Autodesk Fusion 360 part; units mm, degrees
(part 36 of 40)
  line L9834 (264.7992, 181.2097) -> (264.9001, 181.2807) construction
  line L9835 (264.9001, 181.2807) -> (265.0226, 181.3748) construction
  line L9836 (265.0226, 181.3748) -> (265.1426, 181.4727) construction
  line L9837 (265.1426, 181.4727) -> (265.2609, 181.5729) construction
  line L9838 (265.2609, 181.5729) -> (265.3784, 181.6744) construction
  line L9839 (265.3784, 181.6744) -> (265.4954, 181.7767) construction
  line L9840 (265.4954, 181.7767) -> (265.6117, 181.88) construction
  line L9841 (265.6117, 181.88) -> (265.7271, 181.9844) construction
  line L9842 (265.7271, 181.9844) -> (265.8414, 182.0903) construction
  line L9843 (265.8414, 182.0903) -> (265.9544, 182.1981) construction
  line L9844 (265.9544, 182.1981) -> (266.066, 182.3077) construction
  line L9845 (266.066, 182.3077) -> (266.1764, 182.419) construction
  line L9846 (266.1764, 182.419) -> (266.2857, 182.5316) construction
  line L9847 (266.2857, 182.5316) -> (266.3942, 182.6455) construction
  line L9848 (266.3942, 182.6455) -> (266.5018, 182.7603) construction
  line L9849 (266.5018, 182.7603) -> (266.6087, 182.876) construction
  line L9850 (266.6087, 182.876) -> (266.7148, 182.9927) construction
  line L9851 (266.7148, 182.9927) -> (266.8201, 183.1105) construction
  line L9852 (266.8201, 183.1105) -> (266.9246, 183.2292) construction
  line L9853 (266.9246, 183.2292) -> (267.0281, 183.3491) construction
  line L9854 (267.0281, 183.3491) -> (267.1308, 183.47) construction
  line L9855 (267.1308, 183.47) -> (267.2327, 183.5919) construction
  line L9856 (267.2327, 183.5919) -> (267.3337, 183.7148) construction
  line L9857 (267.3337, 183.7148) -> (267.434, 183.8386) construction
  line L9858 (267.434, 183.8386) -> (267.5335, 183.9633) construction
  line L9859 (267.5335, 183.9633) -> (267.6323, 184.0888) construction
  line L9860 (267.6323, 184.0888) -> (267.7304, 184.2151) construction
  line L9861 (267.7304, 184.2151) -> (267.8277, 184.3423) construction
  line L9862 (267.8277, 184.3423) -> (267.9243, 184.4703) construction
  line L9863 (267.9243, 184.4703) -> (268.0201, 184.5991) construction
  line L9864 (268.0201, 184.5991) -> (268.1152, 184.7288) construction
  line L9865 (268.1152, 184.7288) -> (268.2096, 184.8592) construction
  line L9866 (268.2096, 184.8592) -> (268.3032, 184.9905) construction
  line L9867 (268.3032, 184.9905) -> (268.3962, 185.1224) construction
  line L9868 (268.3962, 185.1224) -> (268.4884, 185.2552) construction
  line L9869 (268.4884, 185.2552) -> (268.58, 185.3886) construction
  line L9870 (268.58, 185.3886) -> (268.6708, 185.5228) construction
  line L9871 (268.6708, 185.5228) -> (268.761, 185.6577) construction
  line L9872 (268.761, 185.6577) -> (268.8505, 185.7933) construction
  line L9873 (268.8505, 185.7933) -> (268.9393, 185.9295) construction
  line L9874 (268.9393, 185.9295) -> (269.0275, 186.0665) construction
  line L9875 (269.0275, 186.0665) -> (269.1149, 186.2042) construction
  line L9876 (269.1149, 186.2042) -> (269.2017, 186.3425) construction
  line L9877 (269.2017, 186.3425) -> (269.2878, 186.4815) construction
  line L9878 (269.2878, 186.4815) -> (269.3733, 186.6211) construction
  line L9879 (269.3733, 186.6211) -> (269.4581, 186.7614) construction
  line L9880 (269.4581, 186.7614) -> (269.5422, 186.9023) construction
  line L9881 (269.5422, 186.9023) -> (269.6257, 187.0438) construction
  line L9882 (269.6257, 187.0438) -> (269.7085, 187.186) construction
  line L9883 (269.7085, 187.186) -> (269.7907, 187.3288) construction
  line L9884 (269.7907, 187.3288) -> (269.8723, 187.4721) construction
  line L9885 (269.8723, 187.4721) -> (269.9532, 187.6161) construction
  line L9886 (269.9532, 187.6161) -> (270.0334, 187.7607) construction
  line L9887 (270.0334, 187.7607) -> (270.113, 187.9058) construction
  line L9888 (270.113, 187.9058) -> (270.192, 188.0515) construction
  line L9889 (270.192, 188.0515) -> (270.2703, 188.1978) construction
  line L9890 (270.2703, 188.1978) -> (270.348, 188.3447) construction
  line L9891 (270.348, 188.3447) -> (270.4251, 188.4921) construction
  line L9892 (270.4251, 188.4921) -> (270.5015, 188.6401) construction
  line L9893 (270.5015, 188.6401) -> (270.5773, 188.7886) construction
  line L9894 (270.5773, 188.7886) -> (270.6525, 188.9377) construction
  line L9895 (270.6525, 188.9377) -> (270.727, 189.0873) construction
  line L9896 (270.727, 189.0873) -> (270.801, 189.2374) construction
  line L9897 (270.801, 189.2374) -> (270.8743, 189.3881) construction
  line L9898 (270.8743, 189.3881) -> (270.9469, 189.5393) construction
  line L9899 (270.9469, 189.5393) -> (271.019, 189.6909) construction
  line L9900 (271.019, 189.6909) -> (271.0904, 189.8431) construction
  line L9901 (271.0904, 189.8431) -> (271.1471, 189.9653) construction
  line L9902 (271.1471, 189.9653) -> (271.1893, 190.0572) construction
  line L9903 (271.1893, 190.0572) -> (271.2173, 190.1185) construction
  line L9904 (271.2173, 190.1185) -> (271.2313, 190.1492) construction
  arc A254 (283.5435, 147.7437) -> (283.5435, 152.2563) centre (212.132, 150) ccw
  spline S132 degree 5 poles (257.9473, 109.6737) (257.9705, 109.6533) (258.0174, 109.6132) (258.0893, 109.5549) (258.188, 109.4808) (258.3153, 109.3934) (258.4455, 109.3096) (258.5774, 109.228) (258.7102, 109.1476) (258.8437, 109.068) (258.9778, 108.9893) (259.1127, 108.9117) (259.2488, 108.8358) (259.3863, 108.7617) (259.525, 108.6894) (259.6649, 108.6187) (259.8058, 108.5496) (259.9476, 108.4816) (260.0901, 108.4147) (260.2332, 108.3488) (260.377, 108.284) (260.5215, 108.2202) (260.6667, 108.1576) (260.8127, 108.0961) (260.9594, 108.0358) (261.1069, 107.9766) (261.255, 107.9185) (261.4037, 107.8614) (261.553, 107.8053) (261.7029, 107.7501) (261.8534, 107.6959) (262.0044, 107.6426) (262.156, 107.5903) (262.3081, 107.539) (262.4608, 107.4886) (262.614, 107.4392) (262.7678, 107.3906) (262.922, 107.343) (263.0767, 107.2963) (263.2319, 107.2505) (263.3876, 107.2055) (263.5438, 107.1614) (263.7004, 107.1182) (263.8575, 107.0759) (264.015, 107.0344) (264.1729, 106.9937) (264.3313, 106.9539) (264.4901, 106.915) (264.6493, 106.8769) (264.8089, 106.8396) (264.9689, 106.8031) (265.1293, 106.7674) (265.2901, 106.7326) (265.4513, 106.6985) (265.6129, 106.6653) (265.7748, 106.6328) (265.9371, 106.6012) (266.0997, 106.5703) (266.2627, 106.5403) (266.426, 106.511) (266.5897, 106.4825) (266.7537, 106.4547) (266.9181, 106.4277) (267.0828, 106.4016) (267.2478, 106.3761) (267.4131, 106.3514) (267.5787, 106.3275) (267.7446, 106.3044) (267.9109, 106.282) (268.0774, 106.2603) (268.2442, 106.2394) (268.3779, 106.2233) (268.4783, 106.2115) (268.5453, 106.2038) (268.5789, 106.2) knots 0 0 0 0 0 0 0.01428571 0.02857143 0.04285714 0.05714286 0.07142857 0.08571429 0.1 0.11428571 0.12857143 0.14285714 0.15714286 0.17142857 0.18571429 0.2 0.21428571 0.22857143 0.24285714 0.25714286 0.27142857 0.28571429 0.3 0.31428571 0.32857143 0.34285714 0.35714286 0.37142857 0.38571429 0.4 0.41428571 0.42857143 0.44285714 0.45714286 0.47142857 0.48571429 0.5 0.51428571 0.52857143 0.54285714 0.55714286 0.57142857 0.58571429 0.6 0.61428571 0.62857143 0.64285714 0.65714286 0.67142857 0.68571429 0.7 0.71428571 0.72857143 0.74285714 0.75714286 0.77142857 0.78571429 0.8 0.81428571 0.82857143 0.84285714 0.85714286 0.87142857 0.88571429 0.9 0.91428571 0.92857143 0.94285714 0.95714286 0.97142857 0.98571429 1 1 1 1 1 1
  line L9905 (257.9473, 109.6737) -> (257.9705, 109.6533) construction
  line L9906 (257.9705, 109.6533) -> (258.0174, 109.6132) construction
  line L9907 (258.0174, 109.6132) -> (258.0893, 109.5549) construction
  line L9908 (258.0893, 109.5549) -> (258.188, 109.4808) construction
  line L9909 (258.188, 109.4808) -> (258.3153, 109.3934) construction
  line L9910 (258.3153, 109.3934) -> (258.4455, 109.3096) construction
  line L9911 (258.4455, 109.3096) -> (258.5774, 109.228) construction
  line L9912 (258.5774, 109.228) -> (258.7102, 109.1476) construction
  line L9913 (258.7102, 109.1476) -> (258.8437, 109.068) construction
  line L9914 (258.8437, 109.068) -> (258.9778, 108.9893) construction
  line L9915 (258.9778, 108.9893) -> (259.1127, 108.9117) construction
  line L9916 (259.1127, 108.9117) -> (259.2488, 108.8358) construction
  line L9917 (259.2488, 108.8358) -> (259.3863, 108.7617) construction
  line L9918 (259.3863, 108.7617) -> (259.525, 108.6894) construction
  line L9919 (259.525, 108.6894) -> (259.6649, 108.6187) construction
  line L9920 (259.6649, 108.6187) -> (259.8058, 108.5496) construction
  line L9921 (259.8058, 108.5496) -> (259.9476, 108.4816) construction
  line L9922 (259.9476, 108.4816) -> (260.0901, 108.4147) construction
  line L9923 (260.0901, 108.4147) -> (260.2332, 108.3488) construction
  line L9924 (260.2332, 108.3488) -> (260.377, 108.284) construction
  line L9925 (260.377, 108.284) -> (260.5215, 108.2202) construction
  line L9926 (260.5215, 108.2202) -> (260.6667, 108.1576) construction
  line L9927 (260.6667, 108.1576) -> (260.8127, 108.0961) construction
  line L9928 (260.8127, 108.0961) -> (260.9594, 108.0358) construction
  line L9929 (260.9594, 108.0358) -> (261.1069, 107.9766) construction
  line L9930 (261.1069, 107.9766) -> (261.255, 107.9185) construction
  line L9931 (261.255, 107.9185) -> (261.4037, 107.8614) construction
  line L9932 (261.4037, 107.8614) -> (261.553, 107.8053) construction
  line L9933 (261.553, 107.8053) -> (261.7029, 107.7501) construction
  line L9934 (261.7029, 107.7501) -> (261.8534, 107.6959) construction
  line L9935 (261.8534, 107.6959) -> (262.0044, 107.6426) construction
  line L9936 (262.0044, 107.6426) -> (262.156, 107.5903) construction
  line L9937 (262.156, 107.5903) -> (262.3081, 107.539) construction
  line L9938 (262.3081, 107.539) -> (262.4608, 107.4886) construction
  line L9939 (262.4608, 107.4886) -> (262.614, 107.4392) construction
  line L9940 (262.614, 107.4392) -> (262.7678, 107.3906) construction
  line L9941 (262.7678, 107.3906) -> (262.922, 107.343) construction
  line L9942 (262.922, 107.343) -> (263.0767, 107.2963) construction
  line L9943 (263.0767, 107.2963) -> (263.2319, 107.2505) construction
  line L9944 (263.2319, 107.2505) -> (263.3876, 107.2055) construction
  line L9945 (263.3876, 107.2055) -> (263.5438, 107.1614) construction
  line L9946 (263.5438, 107.1614) -> (263.7004, 107.1182) construction
  line L9947 (263.7004, 107.1182) -> (263.8575, 107.0759) construction
  line L9948 (263.8575, 107.0759) -> (264.015, 107.0344) construction
  line L9949 (264.015, 107.0344) -> (264.1729, 106.9937) construction
  line L9950 (264.1729, 106.9937) -> (264.3313, 106.9539) construction
  line L9951 (264.3313, 106.9539) -> (264.4901, 106.915) construction
  line L9952 (264.4901, 106.915) -> (264.6493, 106.8769) construction
  line L9953 (264.6493, 106.8769) -> (264.8089, 106.8396) construction
  line L9954 (264.8089, 106.8396) -> (264.9689, 106.8031) construction
  line L9955 (264.9689, 106.8031) -> (265.1293, 106.7674) construction
  line L9956 (265.1293, 106.7674) -> (265.2901, 106.7326) construction
  line L9957 (265.2901, 106.7326) -> (265.4513, 106.6985) construction
  line L9958 (265.4513, 106.6985) -> (265.6129, 106.6653) construction
  line L9959 (265.6129, 106.6653) -> (265.7748, 106.6328) construction
  line L9960 (265.7748, 106.6328) -> (265.9371, 106.6012) construction
  line L9961 (265.9371, 106.6012) -> (266.0997, 106.5703) construction
  line L9962 (266.0997, 106.5703) -> (266.2627, 106.5403) construction
  line L9963 (266.2627, 106.5403) -> (266.426, 106.511) construction
  line L9964 (266.426, 106.511) -> (266.5897, 106.4825) construction
  line L9965 (266.5897, 106.4825) -> (266.7537, 106.4547) construction
  line L9966 (266.7537, 106.4547) -> (266.9181, 106.4277) construction
  line L9967 (266.9181, 106.4277) -> (267.0828, 106.4016) construction
  line L9968 (267.0828, 106.4016) -> (267.2478, 106.3761) construction
  line L9969 (267.2478, 106.3761) -> (267.4131, 106.3514) construction
  line L9970 (267.4131, 106.3514) -> (267.5787, 106.3275) construction
  line L9971 (267.5787, 106.3275) -> (267.7446, 106.3044) construction
  line L9972 (267.7446, 106.3044) -> (267.9109, 106.282) construction
  line L9973 (267.9109, 106.282) -> (268.0774, 106.2603) construction
  line L9974 (268.0774, 106.2603) -> (268.2442, 106.2394) construction
  line L9975 (268.2442, 106.2394) -> (268.3779, 106.2233) construction
  line L9976 (268.3779, 106.2233) -> (268.4783, 106.2115) construction
  line L9977 (268.4783, 106.2115) -> (268.5453, 106.2038) construction
  line L9978 (268.5453, 106.2038) -> (268.5789, 106.2) construction
  arc A255 (155.1583, 142.7194) -> (155.697, 139.3184) centre (212.132, 150) ccw
  arc A256 (204.8514, 206.9737) -> (201.4504, 206.435) centre (212.132, 150) ccw
  arc A257 (219.4126, 93.0263) -> (222.8136, 93.565) centre (212.132, 150) ccw
  arc A258 (219.4126, 93.0263) -> (217.6748, 90.8558) centre (219.6661, 91.0425) ccw
  arc A259 (172.7536, 191.8132) -> (170.3188, 189.3784) centre (212.132, 150) ccw
  spline S133 degree 5 poles (206.4369, 89.2315) (206.4341, 89.2007) (206.4291, 89.1391) (206.4242, 89.0467) (206.4223, 88.9234) (206.4264, 88.769) (206.4351, 88.6144) (206.4466, 88.4597) (206.4597, 88.305) (206.4737, 88.1502) (206.4889, 87.9955) (206.5055, 87.8407) (206.524, 87.686) (206.5449, 87.5312) (206.5679, 87.3765) (206.593, 87.2218) (206.6199, 87.0671) (206.6482, 86.9125) (206.6778, 86.7579) (206.7087, 86.6034) (206.7407, 86.4489) (206.7741, 86.2945) (206.8088, 86.1402) (206.8449, 85.986) (206.8823, 85.8318) (206.9211, 85.6778) (206.9611, 85.5238) (207.0023, 85.3699) (207.0447, 85.2161) (207.0881, 85.0624) (207.1327, 84.9088) (207.1784, 84.7553) (207.2252, 84.602) (207.2731, 84.4487) (207.3221, 84.2956) (207.3721, 84.1426) (207.4233, 83.9897) (207.4754, 83.8369) (207.5285, 83.6842) (207.5827, 83.5317) (207.6378, 83.3794) (207.694, 83.2271) (207.751, 83.075) (207.8091, 82.923) (207.8681, 82.7712) (207.9281, 82.6196) (207.989, 82.468) (208.0508, 82.3167) (208.1135, 82.1655) (208.1772, 82.0144) (208.2417, 81.8635) (208.3071, 81.7128) (208.3735, 81.5622) (208.4407, 81.4118) (208.5087, 81.2616) (208.5777, 81.1115) (208.6474, 80.9616) (208.7181, 80.8119) (208.7895, 80.6624) (208.8619, 80.513) (208.935, 80.3638) (209.009, 80.2148) (209.0838, 80.066) (209.1594, 79.9174) (209.2358, 79.7689) (209.313, 79.6207) (209.391, 79.4726) (209.4698, 79.3248) (209.5494, 79.1771) (209.6297, 79.0297) (209.7109, 78.8824) (209.7764, 78.7648) (209.8259, 78.6766) (209.8591, 78.6179) (209.8757, 78.5885) knots 0 0 0 0 0 0 0.01428571 0.02857143 0.04285714 0.05714286 0.07142857 0.08571429 0.1 0.11428571 0.12857143 0.14285714 0.15714286 0.17142857 0.18571429 0.2 0.21428571 0.22857143 0.24285714 0.25714286 0.27142857 0.28571429 0.3 0.31428571 0.32857143 0.34285714 0.35714286 0.37142857 0.38571429 0.4 0.41428571 0.42857143 0.44285714 0.45714286 0.47142857 0.48571429 0.5 0.51428571 0.52857143 0.54285714 0.55714286 0.57142857 0.58571429 0.6 0.61428571 0.62857143 0.64285714 0.65714286 0.67142857 0.68571429 0.7 0.71428571 0.72857143 0.74285714 0.75714286 0.77142857 0.78571429 0.8 0.81428571 0.82857143 0.84285714 0.85714286 0.87142857 0.88571429 0.9 0.91428571 0.92857143 0.94285714 0.95714286 0.97142857 0.98571429 1 1 1 1 1 1
  line L9979 (206.4369, 89.2315) -> (206.4341, 89.2007) construction
  line L9980 (206.4341, 89.2007) -> (206.4291, 89.1391) construction
  line L9981 (206.4291, 89.1391) -> (206.4242, 89.0467) construction
  line L9982 (206.4242, 89.0467) -> (206.4223, 88.9234) construction
  line L9983 (206.4223, 88.9234) -> (206.4264, 88.769) construction
  line L9984 (206.4264, 88.769) -> (206.4351, 88.6144) construction
  line L9985 (206.4351, 88.6144) -> (206.4466, 88.4597) construction
  line L9986 (206.4466, 88.4597) -> (206.4597, 88.305) construction
  line L9987 (206.4597, 88.305) -> (206.4737, 88.1502) construction
  line L9988 (206.4737, 88.1502) -> (206.4889, 87.9955) construction
  line L9989 (206.4889, 87.9955) -> (206.5055, 87.8407) construction
  line L9990 (206.5055, 87.8407) -> (206.524, 87.686) construction
  line L9991 (206.524, 87.686) -> (206.5449, 87.5312) construction
  line L9992 (206.5449, 87.5312) -> (206.5679, 87.3765) construction
  line L9993 (206.5679, 87.3765) -> (206.593, 87.2218) construction
  line L9994 (206.593, 87.2218) -> (206.6199, 87.0671) construction
  line L9995 (206.6199, 87.0671) -> (206.6482, 86.9125) construction
  line L9996 (206.6482, 86.9125) -> (206.6778, 86.7579) construction
  line L9997 (206.6778, 86.7579) -> (206.7087, 86.6034) construction
  line L9998 (206.7087, 86.6034) -> (206.7407, 86.4489) construction
  line L9999 (206.7407, 86.4489) -> (206.7741, 86.2945) construction
  line L10000 (206.7741, 86.2945) -> (206.8088, 86.1402) construction
  line L10001 (206.8088, 86.1402) -> (206.8449, 85.986) construction
  line L10002 (206.8449, 85.986) -> (206.8823, 85.8318) construction
  line L10003 (206.8823, 85.8318) -> (206.9211, 85.6778) construction
  line L10004 (206.9211, 85.6778) -> (206.9611, 85.5238) construction
  line L10005 (206.9611, 85.5238) -> (207.0023, 85.3699) construction
  line L10006 (207.0023, 85.3699) -> (207.0447, 85.2161) construction
  line L10007 (207.0447, 85.2161) -> (207.0881, 85.0624) construction
  line L10008 (207.0881, 85.0624) -> (207.1327, 84.9088) construction
  line L10009 (207.1327, 84.9088) -> (207.1784, 84.7553) construction
  line L10010 (207.1784, 84.7553) -> (207.2252, 84.602) construction
  line L10011 (207.2252, 84.602) -> (207.2731, 84.4487) construction
  line L10012 (207.2731, 84.4487) -> (207.3221, 84.2956) construction
  line L10013 (207.3221, 84.2956) -> (207.3721, 84.1426) construction
  line L10014 (207.3721, 84.1426) -> (207.4233, 83.9897) construction
  line L10015 (207.4233, 83.9897) -> (207.4754, 83.8369) construction
  line L10016 (207.4754, 83.8369) -> (207.5285, 83.6842) construction
  line L10017 (207.5285, 83.6842) -> (207.5827, 83.5317) construction
  line L10018 (207.5827, 83.5317) -> (207.6378, 83.3794) construction
  line L10019 (207.6378, 83.3794) -> (207.694, 83.2271) construction
  line L10020 (207.694, 83.2271) -> (207.751, 83.075) construction
  line L10021 (207.751, 83.075) -> (207.8091, 82.923) construction
  line L10022 (207.8091, 82.923) -> (207.8681, 82.7712) construction
  line L10023 (207.8681, 82.7712) -> (207.9281, 82.6196) construction
  line L10024 (207.9281, 82.6196) -> (207.989, 82.468) construction
  line L10025 (207.989, 82.468) -> (208.0508, 82.3167) construction
  line L10026 (208.0508, 82.3167) -> (208.1135, 82.1655) construction
  line L10027 (208.1135, 82.1655) -> (208.1772, 82.0144) construction
  line L10028 (208.1772, 82.0144) -> (208.2417, 81.8635) construction
  line L10029 (208.2417, 81.8635) -> (208.3071, 81.7128) construction
  line L10030 (208.3071, 81.7128) -> (208.3735, 81.5622) construction
  line L10031 (208.3735, 81.5622) -> (208.4407, 81.4118) construction
  line L10032 (208.4407, 81.4118) -> (208.5087, 81.2616) construction
  line L10033 (208.5087, 81.2616) -> (208.5777, 81.1115) construction
  line L10034 (208.5777, 81.1115) -> (208.6474, 80.9616) construction
  line L10035 (208.6474, 80.9616) -> (208.7181, 80.8119) construction
  line L10036 (208.7181, 80.8119) -> (208.7895, 80.6624) construction
  line L10037 (208.7895, 80.6624) -> (208.8619, 80.513) construction
  line L10038 (208.8619, 80.513) -> (208.935, 80.3638) construction
  line L10039 (208.935, 80.3638) -> (209.009, 80.2148) construction
  line L10040 (209.009, 80.2148) -> (209.0838, 80.066) construction
  line L10041 (209.0838, 80.066) -> (209.1594, 79.9174) construction
  line L10042 (209.1594, 79.9174) -> (209.2358, 79.7689) construction
  line L10043 (209.2358, 79.7689) -> (209.313, 79.6207) construction
  line L10044 (209.313, 79.6207) -> (209.391, 79.4726) construction
  line L10045 (209.391, 79.4726) -> (209.4698, 79.3248) construction
  line L10046 (209.4698, 79.3248) -> (209.5494, 79.1771) construction
  line L10047 (209.5494, 79.1771) -> (209.6297, 79.0297) construction
  line L10048 (209.6297, 79.0297) -> (209.7109, 78.8824) construction
  line L10049 (209.7109, 78.8824) -> (209.7764, 78.7648) construction
  line L10050 (209.7764, 78.7648) -> (209.8259, 78.6766) construction
  line L10051 (209.8259, 78.6766) -> (209.8591, 78.6179) construction
  line L10052 (209.8591, 78.6179) -> (209.8757, 78.5885) construction
  arc A260 (187.6019, 201.9354) -> (188.5839, 204.5366) centre (186.7478, 203.7438) ccw
  arc A261 (239.7302, 200.3721) -> (236.6621, 201.9354) centre (212.132, 150) ccw
  spline S134 degree 5 poles (243.2435, 97.4897) (243.2592, 97.4632) (243.2914, 97.4105) (243.3417, 97.3328) (243.4127, 97.2319) (243.5068, 97.1094) (243.6047, 96.9894) (243.7049, 96.8711) (243.8064, 96.7536) (243.9087, 96.6366) (244.012, 96.5203) (244.1164, 96.4049) (244.2223, 96.2906) (244.3301, 96.1776) (244.4397, 96.066) (244.551, 95.9556) (244.6636, 95.8463) (244.7775, 95.7378) (244.8923, 95.6302) (245.008, 95.5233) (245.1247, 95.4172) (245.2425, 95.3119) (245.3612, 95.2074) (245.4811, 95.1039) (245.602, 95.0012) (245.7239, 94.8993) (245.8468, 94.7983) (245.9706, 94.698) (246.0953, 94.5985) (246.2208, 94.4997) (246.3471, 94.4016) (246.4743, 94.3043) (246.6023, 94.2077) (246.7311, 94.1119) (246.8608, 94.0168) (246.9912, 93.9224) (247.1225, 93.8288) (247.2544, 93.7358) (247.3872, 93.6436) (247.5206, 93.552) (247.6548, 93.4612) (247.7897, 93.371) (247.9253, 93.2815) (248.0615, 93.1927) (248.1985, 93.1045) (248.3362, 93.0171) (248.4745, 92.9303) (248.6135, 92.8442) (248.7531, 92.7587) (248.8934, 92.6739) (249.0343, 92.5898) (249.1758, 92.5063) (249.318, 92.4235) (249.4608, 92.3413) (249.6041, 92.2597) (249.7481, 92.1788) (249.8927, 92.0986) (250.0378, 92.019) (250.1835, 91.94) (250.3298, 91.8617) (250.4767, 91.784) (250.6241, 91.7069) (250.7721, 91.6305) (250.9206, 91.5547) (251.0697, 91.4795) (251.2193, 91.405) (251.3694, 91.331) (251.5201, 91.2577) (251.6713, 91.1851) (251.8229, 91.113) (251.9751, 91.0416) (252.0973, 90.9849) (252.1892, 90.9427) (252.2505, 90.9147) (252.2812, 90.9007) knots 0 0 0 0 0 0 0.01428571 0.02857143 0.04285714 0.05714286 0.07142857 0.08571429 0.1 0.11428571 0.12857143 0.14285714 0.15714286 0.17142857 0.18571429 0.2 0.21428571 0.22857143 0.24285714 0.25714286 0.27142857 0.28571429 0.3 0.31428571 0.32857143 0.34285714 0.35714286 0.37142857 0.38571429 0.4 0.41428571 0.42857143 0.44285714 0.45714286 0.47142857 0.48571429 0.5 0.51428571 0.52857143 0.54285714 0.55714286 0.57142857 0.58571429 0.6 0.61428571 0.62857143 0.64285714 0.65714286 0.67142857 0.68571429 0.7 0.71428571 0.72857143 0.74285714 0.75714286 0.77142857 0.78571429 0.8 0.81428571 0.82857143 0.84285714 0.85714286 0.87142857 0.88571429 0.9 0.91428571 0.92857143 0.94285714 0.95714286 0.97142857 0.98571429 1 1 1 1 1 1
  line L10053 (243.2435, 97.4897) -> (243.2592, 97.4632) construction
  line L10054 (243.2592, 97.4632) -> (243.2914, 97.4105) construction
  line L10055 (243.2914, 97.4105) -> (243.3417, 97.3328) construction
  line L10056 (243.3417, 97.3328) -> (243.4127, 97.2319) construction
  line L10057 (243.4127, 97.2319) -> (243.5068, 97.1094) construction
  line L10058 (243.5068, 97.1094) -> (243.6047, 96.9894) construction
  line L10059 (243.6047, 96.9894) -> (243.7049, 96.8711) construction
  line L10060 (243.7049, 96.8711) -> (243.8064, 96.7536) construction
  line L10061 (243.8064, 96.7536) -> (243.9087, 96.6366) construction
  line L10062 (243.9087, 96.6366) -> (244.012, 96.5203) construction
  line L10063 (244.012, 96.5203) -> (244.1164, 96.4049) construction
  line L10064 (244.1164, 96.4049) -> (244.2223, 96.2906) construction
  line L10065 (244.2223, 96.2906) -> (244.3301, 96.1776) construction
  line L10066 (244.3301, 96.1776) -> (244.4397, 96.066) construction
  line L10067 (244.4397, 96.066) -> (244.551, 95.9556) construction
  line L10068 (244.551, 95.9556) -> (244.6636, 95.8463) construction
  line L10069 (244.6636, 95.8463) -> (244.7775, 95.7378) construction
  line L10070 (244.7775, 95.7378) -> (244.8923, 95.6302) construction
  line L10071 (244.8923, 95.6302) -> (245.008, 95.5233) construction
  line L10072 (245.008, 95.5233) -> (245.1247, 95.4172) construction
  line L10073 (245.1247, 95.4172) -> (245.2425, 95.3119) construction
  line L10074 (245.2425, 95.3119) -> (245.3612, 95.2074) construction
  line L10075 (245.3612, 95.2074) -> (245.4811, 95.1039) construction
  line L10076 (245.4811, 95.1039) -> (245.602, 95.0012) construction
  line L10077 (245.602, 95.0012) -> (245.7239, 94.8993) construction
  line L10078 (245.7239, 94.8993) -> (245.8468, 94.7983) construction
  line L10079 (245.8468, 94.7983) -> (245.9706, 94.698) construction
  line L10080 (245.9706, 94.698) -> (246.0953, 94.5985) construction
  line L10081 (246.0953, 94.5985) -> (246.2208, 94.4997) construction
  line L10082 (246.2208, 94.4997) -> (246.3471, 94.4016) construction
  line L10083 (246.3471, 94.4016) -> (246.4743, 94.3043) construction
  line L10084 (246.4743, 94.3043) -> (246.6023, 94.2077) construction
  line L10085 (246.6023, 94.2077) -> (246.7311, 94.1119) construction
  line L10086 (246.7311, 94.1119) -> (246.8608, 94.0168) construction
  line L10087 (246.8608, 94.0168) -> (246.9912, 93.9224) construction
  line L10088 (246.9912, 93.9224) -> (247.1225, 93.8288) construction
  line L10089 (247.1225, 93.8288) -> (247.2544, 93.7358) construction
  line L10090 (247.2544, 93.7358) -> (247.3872, 93.6436) construction
  line L10091 (247.3872, 93.6436) -> (247.5206, 93.552) construction
  line L10092 (247.5206, 93.552) -> (247.6548, 93.4612) construction
  line L10093 (247.6548, 93.4612) -> (247.7897, 93.371) construction
  line L10094 (247.7897, 93.371) -> (247.9253, 93.2815) construction
  line L10095 (247.9253, 93.2815) -> (248.0615, 93.1927) construction
  line L10096 (248.0615, 93.1927) -> (248.1985, 93.1045) construction
  line L10097 (248.1985, 93.1045) -> (248.3362, 93.0171) construction
  line L10098 (248.3362, 93.0171) -> (248.4745, 92.9303) construction
  line L10099 (248.4745, 92.9303) -> (248.6135, 92.8442) construction
  line L10100 (248.6135, 92.8442) -> (248.7531, 92.7587) construction
  line L10101 (248.7531, 92.7587) -> (248.8934, 92.6739) construction
  line L10102 (248.8934, 92.6739) -> (249.0343, 92.5898) construction
  line L10103 (249.0343, 92.5898) -> (249.1758, 92.5063) construction
  line L10104 (249.1758, 92.5063) -> (249.318, 92.4235) construction
  line L10105 (249.318, 92.4235) -> (249.4608, 92.3413) construction
  line L10106 (249.4608, 92.3413) -> (249.6041, 92.2597) construction
  line L10107 (249.6041, 92.2597) -> (249.7481, 92.1788) construction
  line L10108 (249.7481, 92.1788) -> (249.8927, 92.0986) construction
  line L10109 (249.8927, 92.0986) -> (250.0378, 92.019) construction
  line L10110 (250.0378, 92.019) -> (250.1835, 91.94) construction
  line L10111 (250.1835, 91.94) -> (250.3298, 91.8617) construction
  line L10112 (250.3298, 91.8617) -> (250.4767, 91.784) construction
  line L10113 (250.4767, 91.784) -> (250.6241, 91.7069) construction
  line L10114 (250.6241, 91.7069) -> (250.7721, 91.6305) construction
  line L10115 (250.7721, 91.6305) -> (250.9206, 91.5547) construction
  line L10116 (250.9206, 91.5547) -> (251.0697, 91.4795) construction
  line L10117 (251.0697, 91.4795) -> (251.2193, 91.405) construction
  line L10118 (251.2193, 91.405) -> (251.3694, 91.331) construction
  line L10119 (251.3694, 91.331) -> (251.5201, 91.2577) construction
  line L10120 (251.5201, 91.2577) -> (251.6713, 91.1851) construction
  line L10121 (251.6713, 91.1851) -> (251.8229, 91.113) construction
  line L10122 (251.8229, 91.113) -> (251.9751, 91.0416) construction
  line L10123 (251.9751, 91.0416) -> (252.0973, 90.9849) construction
  line L10124 (252.0973, 90.9849) -> (252.1892, 90.9427) construction
  line L10125 (252.1892, 90.9427) -> (252.2505, 90.9147) construction
  line L10126 (252.2505, 90.9147) -> (252.2812, 90.9007) construction
  spline S135 degree 5 poles (152.5778, 136.6378) (152.5477, 136.631) (152.4876, 136.6167) (152.3982, 136.5929) (152.2803, 136.5565) (152.1347, 136.5049) (151.9904, 136.4489) (151.8468, 136.3901) (151.7037, 136.3299) (151.5609, 136.2687) (151.4184, 136.2065) (151.2763, 136.1429) (151.1349, 136.0774) (150.9941, 136.0098) (150.8541, 135.94) (150.7147, 135.8684) (150.5759, 135.795) (150.4376, 135.7203) (150.2998, 135.6443) (150.1623, 135.5673) (150.0253, 135.4891) (149.8888, 135.4096) (149.7528, 135.3289) (149.6172, 135.247) (149.4822, 135.1637) (149.3477, 135.0792) (149.2136, 134.9936) (149.08, 134.9068) (148.9468, 134.819) (148.814, 134.7302) (148.6817, 134.6403) (148.5499, 134.5494) (148.4185, 134.4575) (148.2875, 134.3646) (148.157, 134.2707) (148.027, 134.1758) (147.8974, 134.08) (147.7682, 133.9832) (147.6394, 133.8854) (147.5111, 133.7868) (147.3832, 133.6873) (147.2558, 133.5869) (147.1288, 133.4856) (147.0022, 133.3834) (146.876, 133.2804) (146.7503, 133.1765) (146.625, 133.0717) (146.5002, 132.9662) (146.3758, 132.8598) (146.2518, 132.7526) (146.1282, 132.6445) (146.0051, 132.5357) (145.8823, 132.4261) (145.7601, 132.3158) (145.6382, 132.2046) (145.5168, 132.0927) (145.3958, 131.98) (145.2752, 131.8665) (145.1551, 131.7523) (145.0354, 131.6374) (144.9161, 131.5218) (144.7973, 131.4054) (144.6789, 131.2882) (144.5609, 131.1704) (144.4433, 131.0519) (144.3262, 130.9326) (144.2095, 130.8127) (144.0932, 130.6921) (143.9774, 130.5707) (143.862, 130.4488) (143.747, 130.3261) (143.6553, 130.2274) (143.5868, 130.1531) (143.5412, 130.1034) (143.5184, 130.0785) knots 0 0 0 0 0 0 0.01428571 0.02857143 0.04285714 0.05714286 0.07142857 0.08571429 0.1 0.11428571 0.12857143 0.14285714 0.15714286 0.17142857 0.18571429 0.2 0.21428571 0.22857143 0.24285714 0.25714286 0.27142857 0.28571429 0.3 0.31428571 0.32857143 0.34285714 0.35714286 0.37142857 0.38571429 0.4 0.41428571 0.42857143 0.44285714 0.45714286 0.47142857 0.48571429 0.5 0.51428571 0.52857143 0.54285714 0.55714286 0.57142857 0.58571429 0.6 0.61428571 0.62857143 0.64285714 0.65714286 0.67142857 0.68571429 0.7 0.71428571 0.72857143 0.74285714 0.75714286 0.77142857 0.78571429 0.8 0.81428571 0.82857143 0.84285714 0.85714286 0.87142857 0.88571429 0.9 0.91428571 0.92857143 0.94285714 0.95714286 0.97142857 0.98571429 1 1 1 1 1 1
  line L10127 (152.5778, 136.6378) -> (152.5477, 136.631) construction
  line L10128 (152.5477, 136.631) -> (152.4876, 136.6167) construction
  line L10129 (152.4876, 136.6167) -> (152.3982, 136.5929) construction
  line L10130 (152.3982, 136.5929) -> (152.2803, 136.5565) construction
  line L10131 (152.2803, 136.5565) -> (152.1347, 136.5049) construction
  line L10132 (152.1347, 136.5049) -> (151.9904, 136.4489) construction
  line L10133 (151.9904, 136.4489) -> (151.8468, 136.3901) construction
  line L10134 (151.8468, 136.3901) -> (151.7037, 136.3299) construction
  line L10135 (151.7037, 136.3299) -> (151.5609, 136.2687) construction
  line L10136 (151.5609, 136.2687) -> (151.4184, 136.2065) construction
  line L10137 (151.4184, 136.2065) -> (151.2763, 136.1429) construction
  line L10138 (151.2763, 136.1429) -> (151.1349, 136.0774) construction
  line L10139 (151.1349, 136.0774) -> (150.9941, 136.0098) construction
  line L10140 (150.9941, 136.0098) -> (150.8541, 135.94) construction
  line L10141 (150.8541, 135.94) -> (150.7147, 135.8684) construction
  line L10142 (150.7147, 135.8684) -> (150.5759, 135.795) construction
  line L10143 (150.5759, 135.795) -> (150.4376, 135.7203) construction
  line L10144 (150.4376, 135.7203) -> (150.2998, 135.6443) construction
  line L10145 (150.2998, 135.6443) -> (150.1623, 135.5673) construction
  line L10146 (150.1623, 135.5673) -> (150.0253, 135.4891) construction
  line L10147 (150.0253, 135.4891) -> (149.8888, 135.4096) construction
  line L10148 (149.8888, 135.4096) -> (149.7528, 135.3289) construction
  line L10149 (149.7528, 135.3289) -> (149.6172, 135.247) construction
  line L10150 (149.6172, 135.247) -> (149.4822, 135.1637) construction
  line L10151 (149.4822, 135.1637) -> (149.3477, 135.0792) construction
  line L10152 (149.3477, 135.0792) -> (149.2136, 134.9936) construction
  line L10153 (149.2136, 134.9936) -> (149.08, 134.9068) construction
  line L10154 (149.08, 134.9068) -> (148.9468, 134.819) construction
  line L10155 (148.9468, 134.819) -> (148.814, 134.7302) construction
  line L10156 (148.814, 134.7302) -> (148.6817, 134.6403) construction
  line L10157 (148.6817, 134.6403) -> (148.5499, 134.5494) construction
  line L10158 (148.5499, 134.5494) -> (148.4185, 134.4575) construction
  line L10159 (148.4185, 134.4575) -> (148.2875, 134.3646) construction
  line L10160 (148.2875, 134.3646) -> (148.157, 134.2707) construction
  line L10161 (148.157, 134.2707) -> (148.027, 134.1758) construction
  line L10162 (148.027, 134.1758) -> (147.8974, 134.08) construction
  line L10163 (147.8974, 134.08) -> (147.7682, 133.9832) construction
  line L10164 (147.7682, 133.9832) -> (147.6394, 133.8854) construction
  line L10165 (147.6394, 133.8854) -> (147.5111, 133.7868) construction
  line L10166 (147.5111, 133.7868) -> (147.3832, 133.6873) construction
  line L10167 (147.3832, 133.6873) -> (147.2558, 133.5869) construction
  line L10168 (147.2558, 133.5869) -> (147.1288, 133.4856) construction
  line L10169 (147.1288, 133.4856) -> (147.0022, 133.3834) construction
  line L10170 (147.0022, 133.3834) -> (146.876, 133.2804) construction
  line L10171 (146.876, 133.2804) -> (146.7503, 133.1765) construction
  line L10172 (146.7503, 133.1765) -> (146.625, 133.0717) construction
  line L10173 (146.625, 133.0717) -> (146.5002, 132.9662) construction
  line L10174 (146.5002, 132.9662) -> (146.3758, 132.8598) construction
  line L10175 (146.3758, 132.8598) -> (146.2518, 132.7526) construction
  line L10176 (146.2518, 132.7526) -> (146.1282, 132.6445) construction
  line L10177 (146.1282, 132.6445) -> (146.0051, 132.5357) construction
  line L10178 (146.0051, 132.5357) -> (145.8823, 132.4261) construction
  line L10179 (145.8823, 132.4261) -> (145.7601, 132.3158) construction
  line L10180 (145.7601, 132.3158) -> (145.6382, 132.2046) construction
  line L10181 (145.6382, 132.2046) -> (145.5168, 132.0927) construction
  line L10182 (145.5168, 132.0927) -> (145.3958, 131.98) construction
  line L10183 (145.3958, 131.98) -> (145.2752, 131.8665) construction
  line L10184 (145.2752, 131.8665) -> (145.1551, 131.7523) construction
  line L10185 (145.1551, 131.7523) -> (145.0354, 131.6374) construction
  line L10186 (145.0354, 131.6374) -> (144.9161, 131.5218) construction
  line L10187 (144.9161, 131.5218) -> (144.7973, 131.4054) construction
  line L10188 (144.7973, 131.4054) -> (144.6789, 131.2882) construction
  line L10189 (144.6789, 131.2882) -> (144.5609, 131.1704) construction
  line L10190 (144.5609, 131.1704) -> (144.4433, 131.0519) construction
  line L10191 (144.4433, 131.0519) -> (144.3262, 130.9326) construction
  line L10192 (144.3262, 130.9326) -> (144.2095, 130.8127) construction
  line L10193 (144.2095, 130.8127) -> (144.0932, 130.6921) construction
  line L10194 (144.0932, 130.6921) -> (143.9774, 130.5707) construction
  line L10195 (143.9774, 130.5707) -> (143.862, 130.4488) construction
  line L10196 (143.862, 130.4488) -> (143.747, 130.3261) construction
  line L10197 (143.747, 130.3261) -> (143.6553, 130.2274) construction
  line L10198 (143.6553, 130.2274) -> (143.5868, 130.1531) construction
  line L10199 (143.5868, 130.1531) -> (143.5412, 130.1034) construction
  line L10200 (143.5412, 130.1034) -> (143.5184, 130.0785) construction
  arc A262 (154.1697, 136.995) -> (155.697, 139.3184) centre (153.7319, 138.9465) ccw
  spline S136 degree 5 poles (156.0975, 125.8052) (156.0692, 125.7929) (156.0122, 125.7692) (155.9258, 125.736) (155.8091, 125.6961) (155.6609, 125.6522) (155.5112, 125.6127) (155.3606, 125.5759) (155.2094, 125.5405) (155.0579, 125.506) (154.906, 125.4726) (154.7537, 125.4406) (154.6008, 125.4104) (154.4472, 125.3824) (154.2929, 125.3565) (154.138, 125.3326) (153.9826, 125.3103) (153.8268, 125.2895) (153.6706, 125.2699) (153.5141, 125.2515) (153.3573, 125.2342) (153.2002, 125.2182) (153.0427, 125.2035) (152.8849, 125.1902) (152.7267, 125.1782) (152.5682, 125.1675) (152.4094, 125.158) (152.2503, 125.1496) (152.0909, 125.1423) (151.9313, 125.1362) (151.7715, 125.1311) (151.6114, 125.1271) (151.4511, 125.1243) (151.2905, 125.1224) (151.1297, 125.1217) (150.9687, 125.122) (150.8075, 125.1234) (150.6461, 125.1258) (150.4845, 125.1292) (150.3227, 125.1335) (150.1608, 125.1389) (149.9986, 125.1452) (149.8363, 125.1525) (149.6739, 125.1608) (149.5113, 125.17) (149.3485, 125.1801) (149.1856, 125.1912) (149.0225, 125.2033) (148.8593, 125.2162) (148.696, 125.23) (148.5325, 125.2448) (148.3689, 125.2604) (148.2052, 125.277) (148.0414, 125.2944) (147.8775, 125.3127) (147.7135, 125.3319) (147.5494, 125.352) (147.3852, 125.3729) (147.2209, 125.3946) (147.0565, 125.4172) (146.892, 125.4407) (146.7274, 125.465) (146.5628, 125.4902) (146.398, 125.5161) (146.2333, 125.5429) (146.0684, 125.5706) (145.9035, 125.599) (145.7385, 125.6282) (145.5735, 125.6583) (145.4084, 125.6892) (145.2433, 125.7208) (145.1112, 125.7468) (145.0121, 125.7666) (144.946, 125.78) (144.9129, 125.7868) knots 0 0 0 0 0 0 0.01428571 0.02857143 0.04285714 0.05714286 0.07142857 0.08571429 0.1 0.11428571 0.12857143 0.14285714 0.15714286 0.17142857 0.18571429 0.2 0.21428571 0.22857143 0.24285714 0.25714286 0.27142857 0.28571429 0.3 0.31428571 0.32857143 0.34285714 0.35714286 0.37142857 0.38571429 0.4 0.41428571 0.42857143 0.44285714 0.45714286 0.47142857 0.48571429 0.5 0.51428571 0.52857143 0.54285714 0.55714286 0.57142857 0.58571429 0.6 0.61428571 0.62857143 0.64285714 0.65714286 0.67142857 0.68571429 0.7 0.71428571 0.72857143 0.74285714 0.75714286 0.77142857 0.78571429 0.8 0.81428571 0.82857143 0.84285714 0.85714286 0.87142857 0.88571429 0.9 0.91428571 0.92857143 0.94285714 0.95714286 0.97142857 0.98571429 1 1 1 1 1 1
  line L10201 (156.0975, 125.8052) -> (156.0692, 125.7929) construction
  line L10202 (156.0692, 125.7929) -> (156.0122, 125.7692) construction
  line L10203 (156.0122, 125.7692) -> (155.9258, 125.736) construction
  line L10204 (155.9258, 125.736) -> (155.8091, 125.6961) construction
  line L10205 (155.8091, 125.6961) -> (155.6609, 125.6522) construction
  line L10206 (155.6609, 125.6522) -> (155.5112, 125.6127) construction
  line L10207 (155.5112, 125.6127) -> (155.3606, 125.5759) construction
  line L10208 (155.3606, 125.5759) -> (155.2094, 125.5405) construction
  line L10209 (155.2094, 125.5405) -> (155.0579, 125.506) construction
  line L10210 (155.0579, 125.506) -> (154.906, 125.4726) construction
  line L10211 (154.906, 125.4726) -> (154.7537, 125.4406) construction
  line L10212 (154.7537, 125.4406) -> (154.6008, 125.4104) construction
  line L10213 (154.6008, 125.4104) -> (154.4472, 125.3824) construction
  line L10214 (154.4472, 125.3824) -> (154.2929, 125.3565) construction
  line L10215 (154.2929, 125.3565) -> (154.138, 125.3326) construction
  line L10216 (154.138, 125.3326) -> (153.9826, 125.3103) construction
  line L10217 (153.9826, 125.3103) -> (153.8268, 125.2895) construction
  line L10218 (153.8268, 125.2895) -> (153.6706, 125.2699) construction
  line L10219 (153.6706, 125.2699) -> (153.5141, 125.2515) construction
  line L10220 (153.5141, 125.2515) -> (153.3573, 125.2342) construction
  line L10221 (153.3573, 125.2342) -> (153.2002, 125.2182) construction
  line L10222 (153.2002, 125.2182) -> (153.0427, 125.2035) construction
  line L10223 (153.0427, 125.2035) -> (152.8849, 125.1902) construction
  line L10224 (152.8849, 125.1902) -> (152.7267, 125.1782) construction
  line L10225 (152.7267, 125.1782) -> (152.5682, 125.1675) construction
  line L10226 (152.5682, 125.1675) -> (152.4094, 125.158) construction
  line L10227 (152.4094, 125.158) -> (152.2503, 125.1496) construction
  line L10228 (152.2503, 125.1496) -> (152.0909, 125.1423) construction
  line L10229 (152.0909, 125.1423) -> (151.9313, 125.1362) construction
  line L10230 (151.9313, 125.1362) -> (151.7715, 125.1311) construction
  line L10231 (151.7715, 125.1311) -> (151.6114, 125.1271) construction
  line L10232 (151.6114, 125.1271) -> (151.4511, 125.1243) construction
  line L10233 (151.4511, 125.1243) -> (151.2905, 125.1224) construction
  line L10234 (151.2905, 125.1224) -> (151.1297, 125.1217) construction
  line L10235 (151.1297, 125.1217) -> (150.9687, 125.122) construction
  line L10236 (150.9687, 125.122) -> (150.8075, 125.1234) construction
  line L10237 (150.8075, 125.1234) -> (150.6461, 125.1258) construction
  line L10238 (150.6461, 125.1258) -> (150.4845, 125.1292) construction
  line L10239 (150.4845, 125.1292) -> (150.3227, 125.1335) construction
  line L10240 (150.3227, 125.1335) -> (150.1608, 125.1389) construction
  line L10241 (150.1608, 125.1389) -> (149.9986, 125.1452) construction
  line L10242 (149.9986, 125.1452) -> (149.8363, 125.1525) construction
  line L10243 (149.8363, 125.1525) -> (149.6739, 125.1608) construction
  line L10244 (149.6739, 125.1608) -> (149.5113, 125.17) construction
  line L10245 (149.5113, 125.17) -> (149.3485, 125.1801) construction
  line L10246 (149.3485, 125.1801) -> (149.1856, 125.1912) construction
  line L10247 (149.1856, 125.1912) -> (149.0225, 125.2033) construction
  line L10248 (149.0225, 125.2033) -> (148.8593, 125.2162) construction
  line L10249 (148.8593, 125.2162) -> (148.696, 125.23) construction
  line L10250 (148.696, 125.23) -> (148.5325, 125.2448) construction
  line L10251 (148.5325, 125.2448) -> (148.3689, 125.2604) construction
  line L10252 (148.3689, 125.2604) -> (148.2052, 125.277) construction
  line L10253 (148.2052, 125.277) -> (148.0414, 125.2944) construction
  line L10254 (148.0414, 125.2944) -> (147.8775, 125.3127) construction
  line L10255 (147.8775, 125.3127) -> (147.7135, 125.3319) construction
  line L10256 (147.7135, 125.3319) -> (147.5494, 125.352) construction
  line L10257 (147.5494, 125.352) -> (147.3852, 125.3729) construction
  line L10258 (147.3852, 125.3729) -> (147.2209, 125.3946) construction
  line L10259 (147.2209, 125.3946) -> (147.0565, 125.4172) construction
  line L10260 (147.0565, 125.4172) -> (146.892, 125.4407) construction
  line L10261 (146.892, 125.4407) -> (146.7274, 125.465) construction
  line L10262 (146.7274, 125.465) -> (146.5628, 125.4902) construction
  line L10263 (146.5628, 125.4902) -> (146.398, 125.5161) construction
  line L10264 (146.398, 125.5161) -> (146.2333, 125.5429) construction
  line L10265 (146.2333, 125.5429) -> (146.0684, 125.5706) construction
  line L10266 (146.0684, 125.5706) -> (145.9035, 125.599) construction
  line L10267 (145.9035, 125.599) -> (145.7385, 125.6282) construction
  line L10268 (145.7385, 125.6282) -> (145.5735, 125.6583) construction
  line L10269 (145.5735, 125.6583) -> (145.4084, 125.6892) construction
  line L10270 (145.4084, 125.6892) -> (145.2433, 125.7208) construction
  line L10271 (145.2433, 125.7208) -> (145.1112, 125.7468) construction
  line L10272 (145.1112, 125.7468) -> (145.0121, 125.7666) construction
  line L10273 (145.0121, 125.7666) -> (144.946, 125.78) construction
  line L10274 (144.946, 125.78) -> (144.9129, 125.7868) construction
  arc A263 (236.3452, 217.2191) -> (232.0535, 218.6136) centre (212.132, 150) ccw
  arc A264 (253.9452, 189.3784) -> (251.5104, 191.8132) centre (212.132, 150) ccw
  spline S137 degree 5 poles (181.0205, 202.5103) (181.0048, 202.5368) (180.9726, 202.5895) (180.9223, 202.6672) (180.8513, 202.7681) (180.7572, 202.8906) (180.6593, 203.0106) (180.5591, 203.1289) (180.4576, 203.2464) (180.3553, 203.3634) (180.252, 203.4797) (180.1476, 203.5951) (180.0417, 203.7094) (179.9339, 203.8224) (179.8243, 203.934) (179.713, 204.0444) (179.6004, 204.1537) (179.4865, 204.2622) (179.3717, 204.3698) (179.256, 204.4767) (179.1393, 204.5828) (179.0215, 204.6881) (178.9028, 204.7926) (178.7829, 204.8961) (178.662, 204.9988) (178.5401, 205.1007) (178.4172, 205.2017) (178.2934, 205.302) (178.1687, 205.4015) (178.0432, 205.5003) (177.9169, 205.5984) (177.7897, 205.6957) (177.6617, 205.7923) (177.5329, 205.8881) (177.4032, 205.9832) (177.2728, 206.0776) (177.1415, 206.1712) (177.0096, 206.2642) (176.8768, 206.3564) (176.7434, 206.448) (176.6092, 206.5388) (176.4743, 206.629) (176.3387, 206.7185) (176.2025, 206.8073) (176.0655, 206.8955) (175.9278, 206.9829) (175.7895, 207.0697) (175.6505, 207.1558) (175.5109, 207.2413) (175.3706, 207.3261) (175.2297, 207.4102) (175.0882, 207.4937) (174.946, 207.5765) (174.8032, 207.6587) (174.6599, 207.7403) (174.5159, 207.8212) (174.3713, 207.9014) (174.2262, 207.981) (174.0805, 208.06) (173.9342, 208.1383) (173.7873, 208.216) (173.6399, 208.2931) (173.4919, 208.3695) (173.3434, 208.4453) (173.1943, 208.5205) (173.0447, 208.595) (172.8946, 208.669) (172.7439, 208.7423) (172.5927, 208.8149) (172.4411, 208.887) (172.2889, 208.9584) (172.1667, 209.0151) (172.0748, 209.0573) (172.0135, 209.0853) (171.9828, 209.0993) knots 0 0 0 0 0 0 0.01428571 0.02857143 0.04285714 0.05714286 0.07142857 0.08571429 0.1 0.11428571 0.12857143 0.14285714 0.15714286 0.17142857 0.18571429 0.2 0.21428571 0.22857143 0.24285714 0.25714286 0.27142857 0.28571429 0.3 0.31428571 0.32857143 0.34285714 0.35714286 0.37142857 0.38571429 0.4 0.41428571 0.42857143 0.44285714 0.45714286 0.47142857 0.48571429 0.5 0.51428571 0.52857143 0.54285714 0.55714286 0.57142857 0.58571429 0.6 0.61428571 0.62857143 0.64285714 0.65714286 0.67142857 0.68571429 0.7 0.71428571 0.72857143 0.74285714 0.75714286 0.77142857 0.78571429 0.8 0.81428571 0.82857143 0.84285714 0.85714286 0.87142857 0.88571429 0.9 0.91428571 0.92857143 0.94285714 0.95714286 0.97142857 0.98571429 1 1 1 1 1 1
  line L10275 (181.0205, 202.5103) -> (181.0048, 202.5368) construction
  line L10276 (181.0048, 202.5368) -> (180.9726, 202.5895) construction
  line L10277 (180.9726, 202.5895) -> (180.9223, 202.6672) construction
  line L10278 (180.9223, 202.6672) -> (180.8513, 202.7681) construction
  line L10279 (180.8513, 202.7681) -> (180.7572, 202.8906) construction
  line L10280 (180.7572, 202.8906) -> (180.6593, 203.0106) construction
  line L10281 (180.6593, 203.0106) -> (180.5591, 203.1289) construction
  line L10282 (180.5591, 203.1289) -> (180.4576, 203.2464) construction
  line L10283 (180.4576, 203.2464) -> (180.3553, 203.3634) construction
  line L10284 (180.3553, 203.3634) -> (180.252, 203.4797) construction
  line L10285 (180.252, 203.4797) -> (180.1476, 203.5951) construction
  line L10286 (180.1476, 203.5951) -> (180.0417, 203.7094) construction
  line L10287 (180.0417, 203.7094) -> (179.9339, 203.8224) construction
  line L10288 (179.9339, 203.8224) -> (179.8243, 203.934) construction
  line L10289 (179.8243, 203.934) -> (179.713, 204.0444) construction
  line L10290 (179.713, 204.0444) -> (179.6004, 204.1537) construction
  line L10291 (179.6004, 204.1537) -> (179.4865, 204.2622) construction
  line L10292 (179.4865, 204.2622) -> (179.3717, 204.3698) construction
  line L10293 (179.3717, 204.3698) -> (179.256, 204.4767) construction
  line L10294 (179.256, 204.4767) -> (179.1393, 204.5828) construction
  line L10295 (179.1393, 204.5828) -> (179.0215, 204.6881) construction
  line L10296 (179.0215, 204.6881) -> (178.9028, 204.7926) construction
  line L10297 (178.9028, 204.7926) -> (178.7829, 204.8961) construction
  line L10298 (178.7829, 204.8961) -> (178.662, 204.9988) construction
  line L10299 (178.662, 204.9988) -> (178.5401, 205.1007) construction
  line L10300 (178.5401, 205.1007) -> (178.4172, 205.2017) construction
  line L10301 (178.4172, 205.2017) -> (178.2934, 205.302) construction
  line L10302 (178.2934, 205.302) -> (178.1687, 205.4015) construction
  line L10303 (178.1687, 205.4015) -> (178.0432, 205.5003) construction
  line L10304 (178.0432, 205.5003) -> (177.9169, 205.5984) construction
  line L10305 (177.9169, 205.5984) -> (177.7897, 205.6957) construction
  line L10306 (177.7897, 205.6957) -> (177.6617, 205.7923) construction
  line L10307 (177.6617, 205.7923) -> (177.5329, 205.8881) construction
  line L10308 (177.5329, 205.8881) -> (177.4032, 205.9832) construction
  line L10309 (177.4032, 205.9832) -> (177.2728, 206.0776) construction
  line L10310 (177.2728, 206.0776) -> (177.1415, 206.1712) construction
  line L10311 (177.1415, 206.1712) -> (177.0096, 206.2642) construction
  line L10312 (177.0096, 206.2642) -> (176.8768, 206.3564) construction
  line L10313 (176.8768, 206.3564) -> (176.7434, 206.448) construction
  line L10314 (176.7434, 206.448) -> (176.6092, 206.5388) construction
  line L10315 (176.6092, 206.5388) -> (176.4743, 206.629) construction
  line L10316 (176.4743, 206.629) -> (176.3387, 206.7185) construction
  line L10317 (176.3387, 206.7185) -> (176.2025, 206.8073) construction
  line L10318 (176.2025, 206.8073) -> (176.0655, 206.8955) construction
  line L10319 (176.0655, 206.8955) -> (175.9278, 206.9829) construction
  line L10320 (175.9278, 206.9829) -> (175.7895, 207.0697) construction
  line L10321 (175.7895, 207.0697) -> (175.6505, 207.1558) construction
  line L10322 (175.6505, 207.1558) -> (175.5109, 207.2413) construction
  line L10323 (175.5109, 207.2413) -> (175.3706, 207.3261) construction
  line L10324 (175.3706, 207.3261) -> (175.2297, 207.4102) construction
  line L10325 (175.2297, 207.4102) -> (175.0882, 207.4937) construction
  line L10326 (175.0882, 207.4937) -> (174.946, 207.5765) construction
  line L10327 (174.946, 207.5765) -> (174.8032, 207.6587) construction
  line L10328 (174.8032, 207.6587) -> (174.6599, 207.7403) construction
  line L10329 (174.6599, 207.7403) -> (174.5159, 207.8212) construction
  line L10330 (174.5159, 207.8212) -> (174.3713, 207.9014) construction
  line L10331 (174.3713, 207.9014) -> (174.2262, 207.981) construction
  line L10332 (174.2262, 207.981) -> (174.0805, 208.06) construction